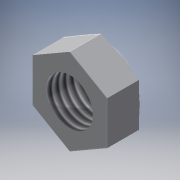
# Autodesk Inventor part: Mutter
Saved by Autodesk Inventor 2016 (Build 200138000, 138)
## iProperties
Created: 2016-04-23
Part Number: Mutter
Material: Generic
Document SubType Name: Modeling
Designer: 3DPrinterUser
Density: 1 g/cm^3
Appearance: Aluminum - Polished
Author: 3DPrinterUser
Autodesk Inventor part; units mm, degrees
ref_plane "YZ Plane" through (0, 0, 0) normal (1, 0, 0) x (0, 1, 0)
ref_plane "XZ Plane" through (0, 0, 0) normal (0, 1, 0) x (-1, 0, 0)
ref_plane "XY Plane" through (0, 0, 0) normal (0, 0, 1) x (1, 0, 0)
sketch "Sketch1" plane through (0, 0, 0) normal (0, 1, 0) x (-1, 0, 0)
  circle A0 centre (0, 0) radius 4
  line L0 (0, -7.5056) -> (-6.5, -3.7528)
  line L1 (-6.5, -3.7528) -> (-6.5, 3.7528)
  line L2 (-6.5, 3.7528) -> (0, 7.5056)
  line L3 (0, 7.5056) -> (6.5, 3.7528)
  line L4 (6.5, 3.7528) -> (6.5, -3.7528)
  line L5 (6.5, -3.7528) -> (0, -7.5056)
  dimension "d0" = 8
  dimension "d1" = 13
  constraints: 12 end point, 2 coincident, 1 centre point, 13 other
  measures "d0" diameter of A0
  measures "d1" distance between parallel lines of L2 L5
extrude "Extrusion1" add sketch "Sketch1" along normal blind 5.5
sketch "Sketch2" plane through (0, 5.5, 0) normal (0, 1, 0) x (1, 0, 0)
  circle A0 centre (0, 0) radius 4 projected
  circle A1 centre (0, 0) radius 6
  dimension "d6" = 2
  constraints: 1 centre point
  measures "d6" radial gap between concentric circles of A0 A1
extrude "Extrusion2" add sketch "Sketch2" along normal blind 1.5
fillet "Fillet1" radius 1.5 2 edges at (-6, 7, 0) (-6, 5.5, 0)
thread "Thread2" size "M8x1.25" class "6H" standard "ANSI Metric M Profile" full length
body "Solid1"
